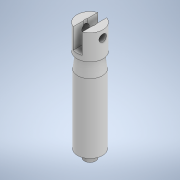
# Autodesk Inventor part: SolenoidShaft
Saved by Autodesk Inventor 2023 (Build 270158000, 158)
## iProperties
Created: 2019-10-21
Part Number: SolenoidShaft
Material: Generic
Document SubType Name: Modeling
Designer: Owner
Density: 1 g/cm^3
Appearance: Default
Author: Owner
Autodesk Inventor part; units mm, degrees
ref_plane "YZ Plane" through (0, 0, 0) normal (1, 0, 0) x (0, 1, 0)
ref_plane "XZ Plane" through (0, 0, 0) normal (0, 1, 0) x (-1, 0, 0)
ref_plane "XY Plane" through (0, 0, 0) normal (0, 0, 1) x (1, 0, 0)
sketch "Sketch1" plane through (0, 0, 0) normal (0, 0, 1) x (1, 0, 0)
  line L0 (2, 45.442) -> (2, -1.498)
  line L1 (2.254, -1.498) -> (3.2702, 1.754)
  line L2 (3.2702, 1.754) -> (4.953, 1.754)
  line L3 (4.953, 1.754) -> (4.953, 29.3765)
  line L4 (4.953, 29.3765) -> (4.2142, 35.3709)
  line L5 (4.2142, 35.3709) -> (5.2137, 35.3709)
  line L6 (5.2137, 35.3709) -> (5.2137, 45.442)
  line L7 (5.2137, 45.442) -> (2, 45.442)
  line L8 (0, 63.454) -> (0, -29.2362) construction
  line L9 (2.7221, 0) -> (1.4605, -4.0372) construction
  line L10 (1.4605, -4.0372) -> (0, -4.0372) construction
  line L11 (2.254, -1.498) -> (2, -1.498)
  point P0 (0, 0)
  dimension "d0" = 2
  dimension "d1" = 4.953
  dimension "d2" = 3.2702
  dimension "d3" = 43.688
  dimension "d4" = 10.0711
  dimension "d5" = 5.9944
  dimension "d16" = 1.4605
  dimension "d17" = 5.7912
  dimension "d18" = 0.254
  constraints: 24 end point, 5 perpendicular, 2 point on line, 2 vertical, 1 collinear, 1 horizontal, 1 horizontal alignment, 1 parallel, 1 vertical alignment
  measures "d0" distance from line of point (0, 0) L0
  measures "d1" distance from line of point (0, 0) L3
  measures "d2" horizontal distance of point (0, 0) L1.end
  measures "d3" distance between parallel lines of L2 L7
  measures "d4" distance of L5.end L6.end
  measures "d5" vertical distance of L5.end L3.end
  measures "d16" distance of L9.end L10.end
  measures "d17" distance between parallel lines of L10 L2
  measures "d18" distance of L1.start L0.end
revolve "Revolution1" add sketch "Sketch1" angle 360 about axis through (0, 63.454, 0) along (0, -1, 0)
sketch "Sketch2" plane through (0, 45.442, 0) normal (0, 1, 0) x (1, 0, 0)
  line L0 (-1.8097, 6.35) -> (1.8097, 6.35)
  line L1 (1.8097, 6.35) -> (1.8097, -6.35)
  line L2 (1.8097, -6.35) -> (-1.8097, -6.35)
  line L3 (-1.8097, -6.35) -> (-1.8097, 6.35)
  point P0 (0, 0)
  point P1 (0, -6.35)
  point P2 (1.8097, 0)
  dimension "d8" = 3.6195
  dimension "d9" = 12.7
  constraints: 8 end point, 2 midpoint, 2 parallel, 1 horizontal, 1 horizontal alignment, 1 perpendicular, 1 vertical alignment
  measures "d8" distance between parallel lines of L1 L3
  measures "d9" distance of L0.end L1.end
extrude "Extrusion1" cut sketch "Sketch2" against normal blind 8.128
sketch "Sketch3" plane through (1.8097, 45.442, 0.8514) normal (-1, 0, 0) x (0, 0, 1)
  circle A0 centre (-0.8514, -2.8829) radius 1.4605
  line L0 (0, 0) -> (4.0382, 0) projected
  point P0 (-0.8514, -45.442)
  dimension "d12" = 2.921
  dimension "d13" = 2.8829
  constraints: 1 centre point
  measures "d12" diameter of A0
  measures "d13" distance from line of L0 A0.centre
extrude "Extrusion2" cut sketch "Sketch3" along normal through all both and the other way through all
body "Solid1"
